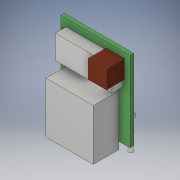
# Autodesk Inventor part: Battery-Management
Saved by Autodesk Inventor 2019 (Build 230136000, 136)
## iProperties
Created: 2018-11-25
Part Number: Battery-Management
Material: Generic
Document SubType Name: Modeling
Designer: lateSWE
Density: 1 g/cm^3
Appearance: Default
Author: lateSWE
Autodesk Inventor part; units mm, degrees
ref_plane "YZ Plane" through (0, 0, 0) normal (1, 0, 0) x (0, 1, 0)
ref_plane "XZ Plane" through (0, 0, 0) normal (0, 1, 0) x (-1, 0, 0)
ref_plane "XY Plane" through (0, 0, 0) normal (0, 0, 1) x (1, 0, 0)
sketch "Sketch1" plane through (0, 0, 0) normal (0, 0, 1) x (1, 0, 0)
  line L0 (0, 0) -> (19, 0)
  line L1 (19, 0) -> (19, 22)
  line L2 (19, 22) -> (0, 22)
  line L3 (0, 22) -> (0, 0)
  dimension "d0" = 19
  dimension "d1" = 22
  constraints: 8 end point, 2 parallel, 1 horizontal, 1 perpendicular
  measures "d0" distance of L2.end L1.end
  measures "d1" distance of L1.end L0.end
extrude "Extrusion1" add sketch "Sketch1" along normal blind 1
sketch "Sketch2" plane through (0, 0, 1) normal (0, 0, 1) x (1, 0, 0)
  line L0 (0, 0) -> (19, 0) projected
  line L1 (0, 0) -> (2.9, 0)
  line L2 (2.9, 0) -> (2.9, 12)
  line L3 (2.9, 12) -> (0, 12)
  line L4 (0, 12) -> (0, 0)
  line L5 (2.9, 12) -> (15.9, 12)
  line L6 (15.9, 12) -> (15.9, -2)
  line L7 (15.9, -2) -> (2.9, -2)
  line L8 (2.9, -2) -> (2.9, 12)
  dimension "d4" = 2.9
  dimension "d5" = 12
  dimension "d6" = 13
  dimension "d7" = 14
  constraints: 16 end point, 4 parallel, 2 horizontal, 2 perpendicular
  measures "d4" distance of L3.end L2.end
  measures "d5" distance of L2.end L1.end
  measures "d6" distance of L6.end L7.end
  measures "d7" distance of L5.end L6.end
extrude "Extrusion2" add sketch "Sketch2" along normal blind 7 contours L2 L5 L6 L0 | L0 L6 L7 L8
sketch "Sketch3" plane through (0, 0, 0) normal (0, 0, -1) x (-1, 0, 0)
  line L0 (-19, 0) -> (-19, 22) projected
  line L1 (-19, 0) -> (-13.5, 0)
  line L2 (-13.5, 0) -> (-13.5, 5)
  line L3 (-13.5, 5) -> (-19, 5)
  line L4 (-19, 5) -> (-19, 0)
  line L5 (-13.5, 0) -> (-5.5, 0)
  line L6 (-5.5, 0) -> (-5.5, 5.5)
  line L7 (-5.5, 5.5) -> (-13.5, 5.5)
  line L8 (-13.5, 5.5) -> (-13.5, 0)
  line L9 (-13.5, 0) -> (-5.5, 0)
  line L10 (-5.5, 0) -> (-5.5, -1.5)
  line L11 (-5.5, -1.5) -> (-13.5, -1.5)
  line L12 (-13.5, -1.5) -> (-13.5, 0)
  point P0 (0, 0)
  dimension "d10" = 5.5
  dimension "d11" = 5
  dimension "d12" = 8
  dimension "d13" = 5.5
  dimension "d16" = 8
  dimension "d17" = 1.5
  constraints: 24 end point, 6 parallel, 3 horizontal, 3 perpendicular
  measures "d10" distance of L3.end L2.end
  measures "d11" distance of L2.end L1.end
  measures "d12" distance of L7.end L6.end
  measures "d13" distance of L6.end L5.end
  measures "d16" distance of L10.end L11.end
  measures "d17" distance of L9.end L10.end
extrude "Extrusion3" add sketch "Sketch3" along normal blind 3 contours L2 L8 L7 L6 L5 | L5 L10 L11 L12
sketch "Sketch4" plane through (0, 0, 1) normal (0, 0, 1) x (1, 0, 0)
  line L0 (19, 22) -> (0, 22) projected
  line L1 (0, 22) -> (1.5, 22)
  line L2 (1.5, 22) -> (1.5, 20.5)
  line L3 (1.5, 20.5) -> (0, 20.5)
  line L4 (0, 20.5) -> (0, 22)
  line L5 (19, 22) -> (17.5, 22)
  line L6 (17.5, 22) -> (17.5, 20.5)
  line L7 (17.5, 20.5) -> (19, 20.5)
  line L8 (19, 20.5) -> (19, 22)
  line L9 (17.5, 20.5) -> (1.5, 20.5)
  line L10 (1.5, 20.5) -> (1.5, 13.5)
  line L11 (1.5, 13.5) -> (17.5, 13.5)
  line L12 (17.5, 13.5) -> (17.5, 20.5)
  point P0 (0, 0)
  dimension "d18" = 1.5
  dimension "d19" = 1.5
  dimension "d20" = 1.5
  dimension "d21" = 1.5
  dimension "d22" = 16
  dimension "d23" = 7
  constraints: 24 end point, 6 parallel, 3 horizontal, 3 perpendicular
  measures "d18" distance of L2.end L3.end
  measures "d19" distance of L1.end L2.end
  measures "d20" distance of L7.end L6.end
  measures "d21" distance of L6.end L5.end
  measures "d22" distance of L11.end L10.end
  measures "d23" distance of L10.end L9.end
extrude "Extrusion4" add sketch "Sketch4" along normal blind 3 contours L12 L11 L10 L9
sketch "Sketch5" plane through (0, 0, 4) normal (0, 0, 1) x (1, 0, 0)
  line L0 (17.5, 20.5) -> (1.5, 20.5) projected
  line L1 (17.5, 20.5) -> (12.5, 20.5)
  line L2 (12.5, 20.5) -> (12.5, 15.5)
  line L3 (12.5, 15.5) -> (17.5, 15.5)
  line L4 (17.5, 15.5) -> (17.5, 20.5)
  point P0 (0, 0)
  dimension "d26" = 5
  dimension "d27" = 5
  constraints: 8 end point, 2 parallel, 1 horizontal, 1 perpendicular
  measures "d26" distance of L3.end L2.end
  measures "d27" distance of L2.end L1.end
extrude "Extrusion5" add sketch "Sketch5" along normal blind 2
sketch "Sketch6" plane through (1.5, 20.5, 1) normal (0, 1, 0) x (1, 0, 0)
  line L0 (0, -3) -> (16, -3) projected
  line L1 (0, -3) -> (11, -3)
  line L2 (11, -3) -> (11, 0)
  line L3 (11, 0) -> (0, 0)
  line L4 (0, 0) -> (0, -3)
  point P0 (-1.5, 1)
  dimension "d30" = 11
  dimension "d31" = 3
  constraints: 8 end point, 2 parallel, 1 horizontal, 1 perpendicular
  measures "d30" distance of L3.end L2.end
  measures "d31" distance of L2.end L1.end
extrude "Extrusion6" cut sketch "Sketch6" against normal blind 0.5
sketch "Sketch7" plane through (17.5, 13.5, 1) normal (1, 0, 0) x (0, 0, -1)
  line L0 (0, 0) -> (-3, 0) projected
  line L1 (-3, 0) -> (0, 0)
  line L2 (0, 0) -> (0, 2)
  line L3 (0, 2) -> (-3, 2)
  line L4 (-3, 2) -> (-3, 0)
  point P0 (1, -13.5)
  dimension "d34" = 3
  dimension "d35" = 2
  constraints: 8 end point, 2 parallel, 1 horizontal, 1 perpendicular
  measures "d34" distance of L3.end L2.end
  measures "d35" distance of L2.end L1.end
extrude "Extrusion7" cut sketch "Sketch7" against normal blind 0.5
sketch "Sketch8" plane through (0, 0, 0) normal (0, 0, -1) x (-1, 0, 0)
  line L0 (-19, 0) -> (-19, 22) projected
  line L1 (-19, 0) -> (-18, 0)
  line L2 (-18, 0) -> (-18, 6)
  line L3 (-18, 6) -> (-19, 6)
  line L4 (-19, 6) -> (-19, 0)
  line L5 (-18, 6) -> (-16.75, 6)
  line L6 (-16.75, 6) -> (-16.75, 5.5)
  line L7 (-16.75, 5.5) -> (-18, 5.5)
  line L8 (-18, 5.5) -> (-18, 6)
  line L9 (-16.75, 5.5) -> (-15.75, 5.5)
  line L10 (-15.75, 5.5) -> (-15.75, 6)
  line L11 (-15.75, 6) -> (-16.75, 6)
  line L12 (-16.75, 6) -> (-16.75, 5.5)
  line L13 (-15.75, 5.5) -> (-14.5, 5.5)
  line L14 (-14.5, 5.5) -> (-14.5, 6)
  line L15 (-14.5, 6) -> (-15.75, 6)
  line L16 (-15.75, 6) -> (-15.75, 5.5)
  line L17 (-13.5, 5.5) -> (-5.5, 5.5) projected
  line L18 (-14.5, 6) -> (-13.5, 6)
  line L19 (-13.5, 6) -> (-13.5, 5.5)
  line L20 (-13.5, 5.5) -> (-14.5, 5.5)
  line L21 (-14.5, 5.5) -> (-14.5, 6)
  point P0 (0, 0)
  dimension "d38" = 1
  dimension "d39" = 6
  dimension "d40" = 1.25
  dimension "d41" = 0.5
  dimension "d42" = 1
  dimension "d43" = 1.25
  dimension "d44" = 1
  dimension "d45" = 0.5
  constraints: 40 end point, 10 parallel, 5 horizontal, 5 perpendicular, 2 point on line
  measures "d38" distance of L3.end L2.end
  measures "d39" distance of L2.end L1.end
  measures "d40" distance of L6.end L7.end
  measures "d41" distance of L5.end L6.end
  measures "d42" distance of L11.end L10.end
  measures "d43" distance of L15.end L14.end
  measures "d44" distance of L17.start L20.end
  measures "d45" distance of L18.end L17.start
extrude "Extrusion8" add sketch "Sketch8" along normal blind 1.5 contours L5 L6 L7 L2 | L15 L14 L13 L10
sketch "Sketch9" plane through (14.5, 6, 0) normal (0, 1, 0) x (1, 0, 0)
  line L0 (1.25, 1.5) -> (0, 1.5) projected
  line L1 (0, 1.5) -> (1.25, 1.5)
  line L2 (1.25, 1.5) -> (1.25, 0)
  line L3 (1.25, 0) -> (0, 0)
  line L4 (0, 0) -> (0, 1.5)
  line L5 (3.5, 1.5) -> (2.25, 1.5) projected
  line L6 (2.25, 1.5) -> (3.5, 1.5)
  line L7 (3.5, 1.5) -> (3.5, 0)
  line L8 (3.5, 0) -> (2.25, 0)
  line L9 (2.25, 0) -> (2.25, 1.5)
  point P0 (-14.5, 0)
  dimension "d48" = 1.25
  dimension "d49" = 1.5
  dimension "d50" = 1.25
  dimension "d51" = 1.5
  constraints: 16 end point, 4 parallel, 2 horizontal, 2 perpendicular
  measures "d48" distance of L2.end L3.end
  measures "d49" distance of L1.end L2.end
  measures "d50" distance of L7.end L8.end
  measures "d51" distance of L6.end L7.end
extrude "Extrusion9" add sketch "Sketch9" along normal blind 0.5
sketch "Sketch10" plane through (16.75, 5.5, 0) normal (0, -1, 0) x (1, 0, 0)
  line L0 (1.25, 0) -> (1.25, -1.5) projected
  line L1 (1.25, -1.5) -> (0.625, -1.5)
  line L2 (0.625, -1.5) -> (0.625, -0.875)
  line L3 (0.625, -0.875) -> (1.25, -0.875)
  line L4 (1.25, -0.875) -> (1.25, -1.5)
  circle A0 centre (0.625, -0.875) radius 0.5
  line L5 (-1, -1.5) -> (-2.25, -1.5) projected
  line L6 (-1, -1.5) -> (-1.625, -1.5)
  line L7 (-1.625, -1.5) -> (-1.625, -0.875)
  line L8 (-1.625, -0.875) -> (-1, -0.875)
  line L9 (-1, -0.875) -> (-1, -1.5)
  circle A1 centre (-1.625, -0.875) radius 0.5
  point P0 (-16.75, 0)
  dimension "d54" = 0.625
  dimension "d55" = 0.625
  dimension "d56" = 1
  dimension "d57" = 0.625
  dimension "d58" = 0.625
  dimension "d59" = 1
  constraints: 16 end point, 4 parallel, 2 centre point, 2 coincident, 2 horizontal, 2 perpendicular
  measures "d54" distance of L2.end L3.end
  measures "d55" distance of L1.end L2.end
  measures "d56" diameter of A0
  measures "d57" distance of L7.end L8.end
  measures "d58" distance of L6.end L7.end
  measures "d59" diameter of A1
extrude "Extrusion10" add sketch "Sketch10" along normal blind 3.5 contours A0 L2 L3 | L3 L2 A0 | A1 L8 L7 | L7 L8 A1
sketch "Sketch11" plane through (17.375, 2, -0.875) normal (0, -1, 0) x (1, 0, 0)
  circle A0 centre (0, 0) radius 0.625
  point P0 (-17.375, 0.875)
  dimension "d62" = 1.25
  constraints: 1 centre point
  measures "d62" diameter of A0
extrude "Extrusion11" add sketch "Sketch11" along normal blind 4.5
body "Solid1"
